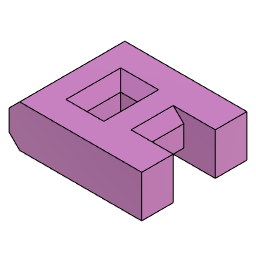
Knotting buckle (Autodesk Fusion 360 design; units mm, degrees)
Autodesk Fusion 360 part; units mm, degrees
sketch "Sketch2" plane through (0, 0, 0) normal (0, 0, 1) x (1, 0, 0)
  line L0 (-2.4, 2.5) -> (2.4, 2.5)
  line L1 (2.4, 2.5) -> (2.4, -2.5)
  line L2 (2.4, -2.5) -> (-2.4, -2.5)
  line L3 (-2.4, -2.5) -> (-2.4, 2.5)
  line L4 (-0.4, -0.8) -> (0.4, -0.8)
  line L5 (0.4, -0.8) -> (0.4, 0.8)
  line L6 (0.4, 0.8) -> (-0.4, 0.8)
  line L7 (-0.4, 0.8) -> (-0.4, -0.8)
  line L8 (0, 2.5) -> (0, -2.5) construction
  line L9 (-0.4, 0) -> (0.4, 0) construction
  line L10 (2.4, 2.5) -> (3.9, 2.5)
  line L11 (3.9, 2.5) -> (3.9, 1)
  line L12 (3.9, 1) -> (2.4, 1)
  line L13 (2.4, 1) -> (2.4, 2.5)
  line L14 (2.4, -2.5) -> (3.9, -2.5)
  line L15 (3.9, -2.5) -> (3.9, -1)
  line L16 (3.9, -1) -> (2.4, -1)
  line L17 (2.4, -1) -> (2.4, -2.5)
  line L18 (2.4, 1) -> (-2.4, 1)
  line L19 (2.4, -1) -> (-2.4, -1)
  dimension "d26" = 1.6
  dimension "d28" = 0.8
  dimension "d38" = 5
  dimension "d41" = 2
  dimension "d42" = 1.5
  dimension "d43" = 1.5
  constraint horizontal L0
  constraint vertical L1
  constraint horizontal L2
  constraint vertical L3
  constraint horizontal L4
  constraint vertical L5
  constraint horizontal L6
  constraint vertical L7
  constraint midpoint origin L8
  constraint midpoint L7 L9.start
  constraint midpoint L5 L9.end
  constraint midpoint origin L9
  constraint vertical L8
  constraint coincident L0 L8.start
  constraint coincident L2 L8.end
  constraint midpoint L0 L8.start
  constraint horizontal L10
  constraint vertical L11
  constraint horizontal L12
  constraint vertical L13
  constraint horizontal L14
  constraint vertical L15
  constraint horizontal L16
  constraint vertical L17
  constraint symmetric L9 L11 L15
  constraint symmetric L9 L12 L16
  constraint coincident L3 L18.end
  constraint perpendicular L3 L18
  constraint perpendicular L1 L19
  constraint coincident L3 L19.end
  measures "d26" distance of L4 L6
  measures "d28" distance of L4.start L4.end
  measures "d38" distance of L0.start L2.end
  measures "d41" distance of L3 L7
  measures "d42" distance of L14.end L15.end
  measures "d43" distance of L1.end L14.end
extrude "Extrude5" add sketch "Sketch2" along normal blind 2
chamfer "Chamfer1" distance 0.5 angle 45 12 edges at (0.4, 0, 0) (-0.4, 0, 0) (0, 0.8, 0) (0, 0.8, 2) (0, -0.8, 0) (0, -0.8, 2) (0.4, 0, 2) (-0.4, 0, 2) (2.4, 0, 0) (2.4, 0, 2) (-2.4, 0, 2) (-2.4, 0, 0)
equation "wire_spacing = 0.8 mm"
